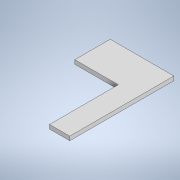
# Autodesk Inventor part: S5_Mainboard
Saved by Autodesk Inventor 2020 (Build 240168000, 168)
## iProperties
Created: 2019-09-06
Part Number: S5_Mainboard
Material: Ogólny
Document SubType Name: Modeling
Designer: atmat
Density: 1 g/cm^3
Appearance: Domyślna
Author: atmat
Autodesk Inventor part; units mm, degrees
ref_plane "YZ Plane" through (0, 0, 0) normal (1, 0, 0) x (0, 1, 0)
ref_plane "XZ Plane" through (0, 0, 0) normal (0, 1, 0) x (-1, 0, 0)
ref_plane "XY Plane" through (0, 0, 0) normal (0, 0, 1) x (1, 0, 0)
sketch "Szkic1" plane through (0, 0, 0) normal (0, 1, 0) x (-1, 0, 0)
  line L0 (34.8855, -22.7009) -> (-28.1145, -22.7009)
  line L1 (-28.1145, -22.7009) -> (-28.1145, -57.7009)
  line L2 (-28.1145, -57.7009) -> (34.8855, -57.7009)
  line L3 (34.8855, -57.7009) -> (34.8855, -22.7009)
  line L4 (-28.1145, -57.7009) -> (-8.1145, -57.7009)
  line L5 (-8.1145, -57.7009) -> (-8.1145, 45.2991)
  line L6 (-8.1145, 45.2991) -> (-28.1145, 45.2991)
  line L7 (-28.1145, 45.2991) -> (-28.1145, -57.7009)
  point P0 (0, 0)
  point P1 (-8.1145, -22.7009)
  dimension "d0" = 63
  dimension "d1" = 35
  dimension "d2" = 103
  dimension "d3" = 20
  constraints: 16 end point, 4 parallel, 2 horizontal, 2 perpendicular
  measures "d0" distance of L1.end L2.end
  measures "d1" distance of L2.end L0.start
  measures "d2" distance of L6.end L1.end
  measures "d3" distance of L5.end L6.end
extrude "Wyciągnięcie proste1" add sketch "Szkic1" along normal blind 4
